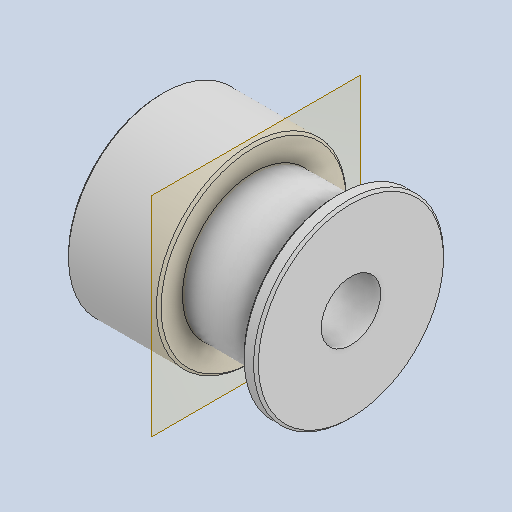
# Autodesk Inventor part: Riemenscheibe
Saved by Autodesk Inventor 2024 (Build 280153000, 153)
## iProperties
Created: 2023-07-28
Part Number: Riemenscheibe
Material: Generisch
Document SubType Name: Modeling
Designer: aewalder
Density: 1 g/cm^3
Appearance: Vorgabe
Author: aewalder
Autodesk Inventor part; units mm, degrees
ref_plane "YZ Plane" through (0, 0, 0) normal (1, 0, 0) x (0, 1, 0)
ref_plane "XZ Plane" through (0, 0, 0) normal (0, 1, 0) x (-1, 0, 0)
ref_plane "XY Plane" through (0, 0, 0) normal (0, 0, 1) x (1, 0, 0)
sketch "Sketch1" plane through (0, 0, 0) normal (0, 0, 1) x (1, 0, 0)
  line L0 (0, 0) -> (0, 8)
  line L1 (0, 8) -> (7.8, 8)
  line L2 (7.8, 8) -> (7.8, 6)
  line L3 (7.8, 6) -> (14.8, 6)
  line L4 (14.8, 6) -> (14.8, 8)
  line L5 (14.8, 8) -> (16, 8)
  line L6 (16, 8) -> (16, 0)
  line L7 (16, 0) -> (0, 0)
  dimension "d0" = 16
  dimension "d1" = 1.2
  dimension "d2" = 7
  dimension "d3" = 16
  dimension "d4" = 12
  constraints: 16 end point, 6 perpendicular, 2 point on line, 1 vertical
  measures "d0" distance between parallel lines of L6 L0
  measures "d1" distance between parallel lines of L6 L4
  measures "d2" distance between parallel lines of L4 L2
  measures "d3" diameter of L1 L7
  measures "d4" diameter of L3 L7
revolve "Revolution1" add sketch "Sketch1" angle 360 about axis through (16, 0, 0) along (-1, 0, 0)
chamfer "Chamfer1" distance 0.2 angle 45 4 edges at (7.8, -8, 0) (0, -8, 0) (14.8, -8, 0) (16, -8, 0)
sketch "Sketch2" plane through (16, 0, 0) normal (1, 0, 0) x (0, 0, -1)
  circle A0 centre (0, 0) radius 2.5
  dimension "d9" = 5
  constraints: 1 centre point, 1 coincident
  measures "d9" diameter of A0
extrude "Extrusion1" cut sketch "Sketch2" against normal through all
ref_plane "Work Plane1" through (8, 0, 0) normal (1, 0, 0) x (0, 0, -1)
body "Solid1"
